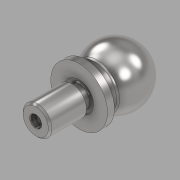
# Autodesk Inventor part: Perilla A01209499ipt
Saved by Autodesk Inventor 2020 (Build 240168000, 168)
## iProperties
Created: 2019-10-11
Part Number: Perilla A01209499ipt
Material: Acero inoxidable
Document SubType Name: Modeling
Designer: gerar
Density: 8 g/cm^3
Appearance: Semipulido
Author: gerar
Autodesk Inventor part; units mm, degrees
ref_plane "YZ Plane" through (0, 0, 0) normal (1, 0, 0) x (0, 1, 0)
ref_plane "XZ Plane" through (0, 0, 0) normal (0, 1, 0) x (-1, 0, 0)
ref_plane "XY Plane" through (0, 0, 0) normal (0, 0, 1) x (1, 0, 0)
sketch "Boceto1" plane through (0, 0, 0) normal (1, 0, 0) x (0, 1, 0)
  line L0 (3.175, 0) -> (3.175, -7.9502)
  line L1 (3.175, -7.9502) -> (2.3622, -7.9502)
  line L2 (2.3622, -7.9502) -> (2.3622, -9.9314)
  line L3 (2.3622, -9.9314) -> (3.175, -9.9314)
  line L4 (3.175, -9.9314) -> (3.175, -9.525)
  line L5 (3.175, -9.525) -> (6.223, -9.525)
  line L6 (6.223, -9.525) -> (6.223, -11.049)
  line L7 (6.223, -11.049) -> (4.7625, -11.049)
  line L8 (0, -30.4355) -> (0, 5.0726) projected
  line L9 (-1.6338, 0) -> (9.8027, 0) construction
  arc A0 (0, -23.8252) -> (4.7625, -13.2751) centre (0, -17.4752) ccw
  line L10 (4.7625, -11.049) -> (4.7625, -13.2751)
  line L11 (3.175, 0) -> (0, 0)
  line L12 (0, 0) -> (0, -23.8252)
  dimension "d0" = 6.35
  dimension "d1" = 12.446
  dimension "d3" = 12.7
  dimension "d4" = 7.9502
  dimension "d5" = 9.525
  dimension "d7" = 17.4752
  dimension "d8" = 11.049
  dimension "d9" = 0.4064
  dimension "d10" = 0.8128
  dimension "d11" = 9.525
  constraints: 22 end point, 8 perpendicular, 3 collinear, 3 point on line, 2 point on circle, 1 centre point, 1 vertical
  measures "d0" diameter of L0 L8
  measures "d1" diameter of L6 L8
  measures "d3" diameter of A0
  measures "d4" distance of L0.start L0.end
  measures "d5" distance between parallel lines of L9 L5
  measures "d7" distance from line of L9 A0.centre
  measures "d8" distance between parallel lines of L9 L7
  measures "d9" distance between parallel lines of L5 L3
  measures "d10" distance between parallel lines of L2 L4
  measures "d11" diameter of L10 L8
revolve "Revolución1" add sketch "Boceto1" angle 360 about axis through (0, 0, -10) along (0, 0, 1)
fillet "Empalme_016" radius 0.4064 2 edges at (0, -2.3622, -9.9314) (0, -3.175, -9.9314)
fillet "Empalme_031" radius 0.7874 2 edges at (0, -4.7625, -11.049) (0, -4.7625, -13.2751)
chamfer "Chaflán1" distance 0.4064 angle 45 1 edges at (0, -3.175, 0) measured on face at (0, -2.675, 0)
sketch "Boceto2" plane through (0, 0, 0) normal (0, 0, 1) x (1, 0, 0)
  point P0 (0, 0)
  point P1 (0, 0)
  constraints: 1 coincident
hole "Agujero1" at (0, 0, 0) direction (0, 0, -1) diameter 2.6416 depth 7.9502 tip angle 118 thread size "6-32 UNC" class "2B" standard "ANSI Unified Screw Threads"
